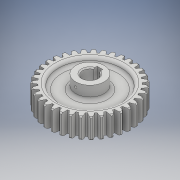
# Autodesk Inventor part: 부품1
Saved by Autodesk Inventor 2018.3 (Build 223284000, 284)
## iProperties
Created: 2019-10-10
Part Number: 부품1
Material: 일반
Document SubType Name: Modeling
Designer: MyTool
Density: 1 g/cm^3
Appearance: 기본값
Author: MyTool
Autodesk Inventor part; units mm, degrees
ref_plane "YZ Plane" through (0, 0, 0) normal (1, 0, 0) x (0, 1, 0)
ref_plane "XZ Plane" through (0, 0, 0) normal (0, 1, 0) x (-1, 0, 0)
ref_plane "XY Plane" through (0, 0, 0) normal (0, 0, 1) x (1, 0, 0)
sketch "스케치1" plane through (0, 0, 0) normal (0, 0, 1) x (1, 0, 0)
  circle A0 centre (0, 0) radius 35 construction
  circle A1 centre (0, 0) radius 37 construction
  circle A2 centre (0, 0) radius 32.5 construction
  line L0 (0.57, 36.9956) -> (0.57, 0) construction
  line L1 (1.57, 34.9648) -> (1.57, 0) construction
  line L2 (2.07, 32.434) -> (2.07, 0) construction
  line L3 (0, 37) -> (0, 0) construction
  arc A3 (2.07, 32.434) -> (0.57, 36.9956) centre (-7.1683, 31.9236) ccw
  arc A4 (-0.57, 36.9956) -> (-2.07, 32.434) centre (7.1683, 31.9236) ccw
  arc A5 (-2.07, 32.434) -> (2.07, 32.434) centre (0, 0) ccw
  arc A6 (0.57, 36.9956) -> (-0.57, 36.9956) centre (0, 0) ccw
  dimension "d0" = 70
  dimension "d2" = 65
  dimension "d1" = 74
  dimension "d3" = 1.57
  dimension "d4" = 1
  dimension "d5" = 0.5
  constraints: 11 point on circle, 8 end point, 5 centre point, 5 coincident, 4 vertical, 3 symmetric about line, 7 other
  measures "d1" diameter of A1
  measures "d3" distance between parallel lines of L1 L3
  measures "d4" distance between parallel lines of L1 L0
  measures "d5" distance between parallel lines of L2 L1
extrude "돌출1" add sketch "스케치1" along normal mid plane 18
chamfer "모따기2" distance 1 angle 45 2 edges at (0, 37, 9) (0, 37, -9)
pattern_circular "원형 패턴1" count 35 over 360 about axis through (0, 0, 0) along (0, 0, 1) of "돌출1", "모따기2"
sketch "스케치2" plane through (0, 0, 9) normal (0, 0, 1) x (1, 0, 0)
  circle A0 centre (0, 0) radius 12.5
  dimension "d11" = 25
  constraints: 1 centre point, 1 coincident
  measures "d11" diameter of A0
extrude "돌출2" add sketch "스케치2" along normal blind 7
sketch "스케치4" plane through (0, 0, 16) normal (0, 0, 1) x (1, 0, 0)
  circle A0 centre (0, 0) radius 6.5
  line L0 (-2.5, 0) -> (2.5, 0)
  line L1 (2.5, 0) -> (2.5, 8.8)
  line L2 (2.5, 8.8) -> (-2.5, 8.8)
  line L3 (-2.5, 8.8) -> (-2.5, 0)
  dimension "d15" = 13
  dimension "d16" = 2.3
  dimension "d17" = 5
  dimension "d18" = 2.5
  constraints: 8 end point, 2 parallel, 1 centre point, 1 coincident, 1 horizontal, 1 perpendicular
  measures "d15" diameter of A0
  measures "d16" distance edge to line of A0 L2
  measures "d17" distance of L1.end L2.end
  measures "d18" distance from line of point (0, 0) L3
extrude "돌출3" cut sketch "스케치4" against normal up to next
chamfer "모따기1" distance 1 angle 45 2 edges at (0, -6.5, 16) (0, -6.5, -9)
sketch "스케치5" plane through (0, 0, 0) normal (0, 1, 0) x (-1, 0, 0)
  circle A0 centre (0, 12) radius 1
  line L0 (12.5, 16) -> (-12.5, 16) projected
  point P0 (0, 0)
  dimension "d25" = 2
  dimension "d26" = 4
  constraints: 1 centre point
  measures "d25" diameter of A0
  measures "d26" distance from line of L0 A0.centre
extrude "돌출4" cut sketch "스케치5" against normal through all
sketch "스케치6" plane through (0, 0, 9) normal (0, 0, 1) x (1, 0, 0)
  circle A0 centre (0, 0) radius 27.5
  circle A1 centre (0, 0) radius 12.5
  dimension "d32" = 55
  dimension "d33" = 25
  constraints: 2 centre point, 2 coincident
  measures "d32" diameter of A0
  measures "d33" diameter of A1
extrude "돌출5" cut sketch "스케치6" against normal blind 5
mirror "미러1" about plane through (0, 0, 0) normal (0, 0, 1) of "돌출5"
fillet "모깎기2" radius 3 6 edges at (-27.5, 0, 9) (-27.5, 0, 4) (-12.5, 0, 4) (-12.5, 0, -4) (-27.5, 0, -4) (-27.5, 0, -9)
